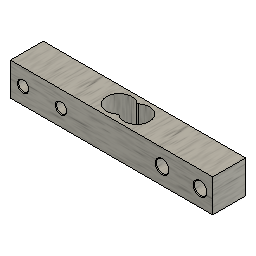
Loadcell_5kg (Autodesk Fusion 360 design; units mm, degrees)
Autodesk Fusion 360 part; units mm, degrees
note: some values were not read from the file. Set by a fixed rule: which sketch regions a step uses.
sketch "Sketch1" plane through (0, 0, 0) normal (0, 1, 0) x (1, 0, 0) in component "Rod"
  line L0 (-27.9791, 13.5539) -> (52.0209, 13.5539)
  line L1 (52.0209, 13.5539) -> (52.0209, 0.5539)
  line L2 (52.0209, 0.5539) -> (-27.9791, 0.5539)
  line L3 (-27.9791, 0.5539) -> (-27.9791, 13.5539)
  dimension "d1" = 80
  dimension "d2" = 13
  constraint horizontal L0
  constraint vertical L1
  constraint horizontal L2
  constraint vertical L3
  measures "d1" distance of L0.start L0.end
  measures "d2" distance of L0.start L2.end
extrude "Extrude1" add sketch "Sketch1" along normal blind 13 in component "Rod"
sketch "Sketch2" plane through (0, 13, 0) normal (0, 1, 0) x (-1, 0, 0) in component "Rod"
  line L0 (27.9791, -0.5539) -> (-52.0209, -0.5539)
  line L1 (-52.0209, -0.5539) -> (-52.0209, -13.5539)
  line L2 (-52.0209, -13.5539) -> (27.9791, -13.5539)
  line L3 (27.9791, -13.5539) -> (27.9791, -0.5539)
  line L4 (27.9791, -7.0539) -> (-52.0209, -7.0539) construction
  line L5 (-12.0209, -7.0539) -> (-12.0209, -13.5539) construction
  line L6 (-12.0209, -7.0539) -> (-12.0209, -0.5539) construction
  circle A0 centre (-8.5209, -7.0539) radius 5
  circle A1 centre (-15.5209, -7.0539) radius 5
  dimension "d5" = 10
  dimension "d6" = 10
  dimension "d7" = 3.5
  dimension "d8" = 3.5
  constraint midpoint L3 L4.start
  constraint midpoint L1 L4.end
  constraint midpoint L4 L5.start
  constraint midpoint L2 L5.end
  constraint midpoint L0 L6.end
  constraint coincident L4 A0.centre
  constraint coincident L4 A1.centre
  measures "d5" diameter of A0
  measures "d6" diameter of A1
  measures "d7" distance of L5.start A0.centre
  measures "d8" distance of L5.start A1.centre
extrude "Extrude2" cut sketch "Sketch2" against normal blind 13 contours A0 A1 | A0 A1 | A0 A1 in component "Rod"
sketch "Sketch3" plane through (0, 0, -0.5539) normal (0, 0, 1) x (1, 0, 0) in component "Rod"
  line L0 (-27.9791, 0) -> (52.0209, 0)
  line L1 (52.0209, 0) -> (52.0209, 13)
  line L2 (52.0209, 13) -> (-27.9791, 13)
  line L3 (-27.9791, 13) -> (-27.9791, 0)
  line L4 (-27.9791, 6.5) -> (52.0209, 6.5) construction
  circle A0 centre (-22.9791, 6.5) radius 2
  circle A1 centre (-7.9791, 6.5) radius 2
  circle A2 centre (32.0209, 6.5) radius 2.5
  circle A3 centre (47.0209, 6.5) radius 2.5
  line L5 (12.0209, 13) -> (12.0209, 0) construction
  dimension "d11" = 4
  dimension "d12" = 4
  dimension "d13" = 5
  dimension "d14" = 5
  dimension "d15" = 40
  dimension "d16" = 15
  dimension "d17" = 15
  dimension "d18" = 20
  constraint midpoint L3 L4.start
  constraint midpoint L1 L4.end
  constraint coincident L4 A0.centre
  constraint coincident L4 A1.centre
  constraint coincident L4 A2.centre
  constraint coincident L4 A3.centre
  constraint midpoint L2 L5.start
  constraint midpoint L0 L5.end
  measures "d11" diameter of A0
  measures "d12" diameter of A1
  measures "d13" diameter of A2
  measures "d14" diameter of A3
  measures "d15" distance of A1.centre A2.centre
  measures "d16" distance of A2.centre A3.centre
  measures "d17" distance of A0.centre A1.centre
  measures "d18" distance of A2.centre L5
extrude "Extrude3" cut sketch "Sketch3" against normal blind 13 contours A0 | A1 | A2 | A3 in component "Rod"
fillet "Fillet1" radius 0.25 8 edges at (44.6901, 7.404, -0.5539) (29.6901, 7.404, -0.5539) (-9.8437, 7.2232, -0.5539) (-24.8437, 7.2232, -0.5539) (-24.8437, 5.7768, -13.5539) (-9.8437, 5.7768, -13.5539) (29.6901, 5.596, -13.5539) (44.6901, 5.596, -13.5539) in component "Rod"
fillet "Fillet2" radius 0.5 2 edges at (12.0209, 6.5, -3.4831) (12.0209, 6.5, -10.6246) in component "Rod"
component "Rod" placed x (1, 0, 0) y (0, 1, 0) z (0, 0, 1) at (0, 0, 0)
